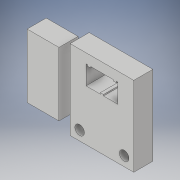
# Autodesk Inventor part: attrape_ball
Saved by Autodesk Inventor 2019 (Build 230136000, 136)
## iProperties
Created: 2018-09-25
Part Number: attrape_ball
Material: Générique
Document SubType Name: Modeling
Designer: Jérémy
Density: 1 g/cm^3
Appearance: Par défaut
Author: Jérémy
Autodesk Inventor part; units mm, degrees
ref_plane "YZ Plane" through (0, 0, 0) normal (1, 0, 0) x (0, 1, 0)
ref_plane "XZ Plane" through (0, 0, 0) normal (0, 1, 0) x (-1, 0, 0)
ref_plane "XY Plane" through (0, 0, 0) normal (0, 0, 1) x (1, 0, 0)
sketch "Esquisse1" plane through (0, 0, 0) normal (0, 0, 1) x (1, 0, 0)
  line L0 (-11.2398, 14.5606) -> (8.7602, 14.5606)
  line L1 (8.7602, 14.5606) -> (8.7602, -10.4394)
  line L2 (-11.2398, -10.4394) -> (-11.2398, 14.5606)
  line L3 (-11.2398, 14.5606) -> (-1.2398, 14.5606) construction
  line L4 (-1.2398, 14.5606) -> (8.7602, 14.5606) construction
  line L5 (-1.2398, 5.1758) -> (-1.2398, -12.1236) construction
  line L6 (-6.2398, 11.5606) -> (3.7602, 11.5606)
  line L7 (3.7602, 11.5606) -> (3.7602, 5.5606)
  line L8 (3.7602, 5.5606) -> (-6.2398, 5.5606)
  line L9 (-6.2398, 5.5606) -> (-6.2398, 11.5606)
  line L10 (-24.7357, 11.7717) -> (-14.7357, 11.7717)
  line L11 (-14.7357, 11.7717) -> (-14.7357, -8.2283)
  line L12 (-14.7357, -8.2283) -> (-24.7357, -8.2283)
  line L13 (-24.7357, -8.2283) -> (-24.7357, 11.7717)
  line L14 (-5.7398, 11.5606) -> (-5.7398, 11.1606)
  line L15 (-5.7398, 11.1606) -> (-4.7398, 11.1606)
  line L16 (-4.7398, 11.1606) -> (-4.7398, 11.5606)
  line L17 (2.2602, 11.5606) -> (2.2602, 11.1606)
  line L18 (2.2602, 11.1606) -> (3.2602, 11.1606)
  line L19 (3.2602, 11.1606) -> (3.2602, 11.5606)
  line L20 (-1.7398, 5.5606) -> (-1.7398, 5.9606)
  line L21 (-1.7398, 5.9606) -> (-0.7398, 5.9606)
  line L22 (-0.7398, 5.9606) -> (-0.7398, 5.5606)
  line L23 (-6.2398, 11.5606) -> (-1.2398, 11.5606) construction
  line L24 (-1.2398, 11.5606) -> (3.7602, 11.5606) construction
  line L25 (-11.2398, -10.4394) -> (8.7602, -10.4394)
  circle A0 centre (-8.2398, -7.4394) radius 1.5
  circle A1 centre (5.7602, -7.4394) radius 1.5
  dimension "d0" = 20
  dimension "d2" = 25
  dimension "d3" = 6
  dimension "d4" = 3
  dimension "d5" = 10
  dimension "d6" = 10
  dimension "d7" = 20
  dimension "d8" = 1
  dimension "d9" = 0.4
  dimension "d10" = 0.4
  dimension "d11" = 0.5
  dimension "d12" = 0.5
  dimension "d13" = 4.5
  dimension "d18" = 3
  dimension "d19" = 3
  dimension "d20" = 3
  constraints: 52 end point, 11 perpendicular, 10 point on line, 6 parallel, 4 equal length, 4 horizontal, 2 centre point, 2 collinear, 2 midpoint, 1 symmetric about line, 1 other
  measures "d0" distance of L2.end L1.start
  measures "d2" distance of L1.start L1.end
  measures "d3" distance of L6.end L7.end
  measures "d4" vertical distance of L2.end L9.end
  measures "d5" distance of L7.end L9.start
  measures "d6" distance of L10.start L11.start
  measures "d7" distance of L13.start L10.start
  measures "d8" distance of L14.end L16.start
  measures "d9" distance of L21.end L22.end
  measures "d10" distance of L14.start L14.end
  measures "d11" horizontal distance of L9.end L14.end
  measures "d12" horizontal distance of L6.end L18.end
  measures "d13" horizontal distance of L9.start L20.end
  measures "d18" diameter of A0
  measures "d19" distance from line of L25 A0.centre
  measures "d20" distance from line of L2 A0.centre
extrude "Extrusion1" add sketch "Esquisse1" along normal blind 6 contours L0 L1 L25 L2 | L6 L16 L15 L14 | L20 L21 L22 L8 | L6 L19 L18 L17 | L10 L11 L12 L13
equation "\"d0\" = L_modules"
equation "\"d3\" = epaisseur_modules"
equation "\"d5\" = 0.5 * d0"
equation "\"d6\" = d5"
equation "\"d8\" = d15"
equation "\"d9\" = d16"
equation "\"d10\" = d16"
equation "\"d11\" = d17"
equation "\"d12\" = d17"
equation "\"d13\" = 0.5 * d5 - 0.5 * d8"
equation "\"d19\" = d20"
equation "\"d21\" = epaisseur_modules"
equation "\"d14\" = 8.2"
equation "\"d15\" = 1"
equation "\"d16\" = 0.4"
equation "\"d17\" = 0.5"
equation "\"epaisseur\" = 6"
equation "\"ecartement\" = 25"
equation "\"dvis\" = 3"
equation "\"largeur\" = 32"
equation "\"L_attache_carte\" = 15"
equation "\"marge_attache_carte\" = 5"
equation "\"L_cubi\" = 81.6"
equation "\"largeur_cubi\" = 81.6"
equation "\"L_moteur\" = 28.3"
equation "\"marge_trou\" = 2"
equation "\"taille_trou\" = 7"
equation "\"H_cubi\" = 81.6"
equation "\"epaisseur_wheel\" = 9"
equation "\"H_nez\" = 25"
equation "\"chanfrein\" = 0.5"
equation "\"H_trou_int\" = 0.5"
equation "\"L_trou_int\" = 1.2"
equation "\"pos_trou_int_1\" = 0.6"
equation "\"pos_trou_int_2\" = 2.9"
equation "\"epaisseur_modules\" = 6"
equation "\"L_modules\" = 20"
equation "\"L_metabois\" = 8.2"
equation "\"epaisseur_metabois\" = 3"
